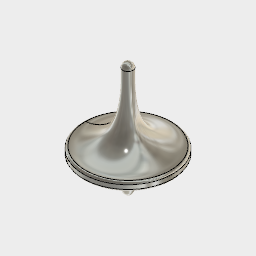
fusion (Autodesk Fusion 360 design; units mm, degrees)
Autodesk Fusion 360 part; units mm, degrees
note: some values were not read from the file. Set by a fixed rule: which sketch regions a step uses.
sketch "Sketch1" plane through (0, 0, 0) normal (0, 1, 0) x (1, 0, 0)
  line L0 (0, -1.75) -> (0, -22.5) construction
  line L1 (-9.4555, -79.9492) -> (9.1952, -79.9492) construction
  line L2 (-30.8196, -29.0673) -> (-30.8196, -32) construction
  spline S0 degree 5 poles (-3.7449, -79.9492) (-3.7093, -78.5922) (-3.6609, -75.9066) (-3.6562, -71.9637) (-3.7924, -66.8887) (-4.2362, -60.9167) (-5.0006, -55.4065) (-6.1321, -50.4535) (-7.6646, -46.1389) (-9.6075, -42.5106) (-11.9295, -39.5587) (-14.5462, -37.196) (-17.346, -35.3013) (-20.2119, -33.7568) (-23.0409, -32.4803) (-25.7707, -31.4716) (-27.8549, -30.9285) (-29.3597, -30.7021) (-30.3372, -30.6369) (-30.8196, -30.6257) knots 0 0 0 0 0 0 0.066667 0.133333 0.2 0.266667 0.333333 0.4 0.466667 0.533333 0.6 0.666667 0.733333 0.8 0.866667 0.933333 1 1 1 1 1 1
  line L3 (-3.9366, -87.2665) -> (-3.5532, -72.6319)
  line L4 (-25.7151, -30.7438) -> (-35.9242, -30.5077)
  arc A0 (-32.3781, -29.0673) -> (-30.8196, -30.6257) centre (-30.8196, -29.0673) ccw
  line L5 (-32.3781, -29.0673) -> (-32.3781, -26.0673)
  line L6 (-32.3781, -27.5673) -> (-30, -27.5673) construction
  arc A1 (-30.8196, -24.5088) -> (-32.3781, -26.0673) centre (-30.8196, -26.0673) ccw
  line L7 (0, -83.6941) -> (0, 0)
  spline S1 degree 5 poles (-30.8196, -24.5088) (-30.3972, -24.3569) (-29.561, -24.0556) (-28.3322, -23.6106) (-26.7452, -23.0313) (-24.8474, -22.3297) (-23.0352, -21.6476) (-21.3071, -20.9787) (-19.6592, -20.3122) (-18.0849, -19.6315) (-16.5738, -18.9126) (-15.1137, -18.1275) (-13.6946, -17.2483) (-12.3114, -16.2513) (-10.9664, -15.1212) (-9.6742, -13.8554) (-8.4593, -12.4657) (-7.3484, -10.9753) (-6.3643, -9.4173) (-5.5189, -7.833) (-4.8066, -6.2702) (-4.1963, -4.782) (-3.6397, -3.4223) (-3.0818, -2.2414) (-2.4704, -1.2811) (-1.7674, -0.5701) (-1.1177, -0.2102) (-0.5789, -0.059) (-0.1968, -0.0109) (0, 0) knots 0 0 0 0 0 0 0.04 0.08 0.12 0.16 0.2 0.24 0.28 0.32 0.36 0.4 0.44 0.48 0.52 0.56 0.6 0.64 0.68 0.72 0.76 0.8 0.84 0.88 0.92 0.96 1 1 1 1 1 1
  arc A2 (-3.7449, -79.9492) -> (0, -83.6941) centre (0, -79.9492) ccw
  point P0 (-9.4555, -43.0689)
  point P1 (-21.1598, -33.3629)
  point P2 (-19.4141, -20.1976)
  point P3 (-11.6697, -15.6906)
  point P4 (-5.4488, -7.6288)
  point P5 (-2.5922, -1.5348)
  dimension "d2" = 3
  measures "d2" distance of A0.start L5.end
revolve "Revolve1" add sketch "Sketch1" angle 360 about axis through (0, 0, 83.6941) along (0, 0, -1)
